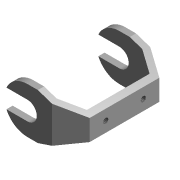
# Autodesk Inventor part: Forearm
Saved by Autodesk Inventor 2011 (Build 150239000, 239)
## iProperties
Created: 2010-11-25
Part Number: Forearm
Document SubType Name: Modeling
Designer: Milton
Density: 1 g/cm^3
Author: Milton
Autodesk Inventor part; units mm, degrees
ref_plane "YZ Plane" through (0, 0, 0) normal (1, 0, 0) x (0, 1, 0)
ref_plane "XZ Plane" through (0, 0, 0) normal (0, 1, 0) x (-1, 0, 0)
ref_plane "XY Plane" through (0, 0, 0) normal (0, 0, 1) x (1, 0, 0)
sketch "Sketch1" plane through (0, 0, 0) normal (0, 0, 1) x (1, 0, 0)
  line L0 (26.057, 23.9046) -> (48.057, 23.9046)
  line L1 (26.057, 64.9046) -> (48.057, 64.9046)
  line L2 (57.057, 59.4046) -> (57.057, 29.4046)
  line L3 (48.057, 23.9046) -> (26.057, 23.9046)
  line L4 (26.057, 23.9046) -> (26.057, 20.9046)
  line L5 (26.057, 20.9046) -> (48.9011, 20.9046)
  line L6 (60.057, 27.7221) -> (60.057, 61.0871)
  line L7 (26.057, 64.9046) -> (26.057, 67.9046)
  line L8 (26.057, 67.9046) -> (48.9011, 67.9046)
  line L9 (57.057, 59.4046) -> (48.057, 64.9046)
  line L10 (60.057, 61.0871) -> (48.9011, 67.9046)
  line L11 (57.057, 29.4046) -> (48.057, 23.9046)
  line L12 (60.057, 27.7221) -> (48.9011, 20.9046)
  point P0 (0, 0)
  dimension "d0" = 3
  dimension "d1" = 3
  dimension "d2" = 3
  dimension "d3" = 34
  dimension "d4" = 34
  dimension "d6" = 41
  dimension "d7" = 9
  dimension "d8" = 5.5
  constraints: 26 end point
  measures "d0" distance of L1.start L7.end
  measures "d1" distance of L0.start L4.end
  measures "d2" distance between parallel lines of L6 L2
  measures "d3" distance between parallel lines of L6 L7
  measures "d4" distance between parallel lines of L6 L4
  measures "d6" distance between parallel lines of L0 L1
  measures "d7" horizontal distance of L2.start L1.end
  measures "d8" vertical distance of L2.start L1.end
extrude "Extrusion1" add sketch "Sketch1" along normal blind 22
sketch "Sketch2" plane through (26.057, 20.9046, 0) normal (0, -1, 0) x (1, 0, 0)
  line L0 (22.8441, 22) -> (0, 22) projected
  line L1 (0, 0) -> (0, 22) projected
  line L2 (0, 0) -> (22.8441, 0) projected
  line L3 (11, 22) -> (-1, 22)
  line L4 (-1, 22) -> (-1, 0)
  line L5 (-1, 0) -> (11, 0)
  line L6 (16, 22) -> (34, 16)
  line L7 (34, 0) -> (34, 22) projected
  line L8 (16, 22) -> (36, 22)
  line L9 (36, 22) -> (36, 0)
  line L10 (36, 0) -> (16, 0)
  line L11 (16, 0) -> (34, 6)
  line L12 (34, 16) -> (34, 6)
  arc A0 (11, 6.5) -> (11, 15.5) centre (11, 11) ccw
  line L13 (11, 15.5) -> (0.9626, 15.5)
  line L14 (11, 6.5) -> (0.9626, 6.5)
  arc A1 (0.9626, 6.5) -> (11, 0) centre (11, 11) ccw
  arc A2 (11, 22) -> (0.9626, 15.5) centre (11, 11) ccw
  point P0 (-26.057, 0)
  dimension "d11" = 11
  dimension "d12" = 12
  dimension "d14" = 6
  dimension "d15" = 6
  dimension "d16" = 18
  dimension "d17" = 18
  dimension "d20" = 9
  constraints: 22 end point, 7 point on line, 6 point on circle, 4 perpendicular, 3 centre point, 2 parallel, 2 tangent, 1 coincident
  measures "d11" distance from line of L1 A1.centre
  measures "d12" distance of L3.start L3.end
  measures "d14" distance from line of L10 L11.end
  measures "d15" distance from line of L8 L6.end
  measures "d16" distance from line of L7 L6.start
  measures "d17" distance from line of L7 L10.end
  measures "d20" diameter of A0
extrude "Extrusion2" cut sketch "Sketch2" against normal through all contours L8 L7 L6 L0 | L8 L9 L10 L7 | A2 L13 A0 L14 A1 L2 L1 L0 | L1 L5 L4 L3 | L7 L10 L2 L11
sketch "Sketch3" plane through (60.057, 27.7221, 6) normal (1, 0, 0) x (0, 0, -1)
  circle A0 centre (-5, 7.6825) radius 1.5 projected
  circle A1 centre (-5, 25.6825) radius 1.5 projected
  circle A2 centre (-5, 25.6825) radius 1.5
  circle A3 centre (-5, 7.6825) radius 1.5
  point P0 (6, -27.7221)
  constraints: 2 centre point, 2 coincident, 2 concentric
hole "Hole1" at (60.057, 35.4046, 11) at (60.057, 53.4046, 11) direction (-1, 0, 0) diameter 2.459 end through all thread size "M3x0.5" class "6H" standard "ANSI Metric M Profile"
body "Solid1"
